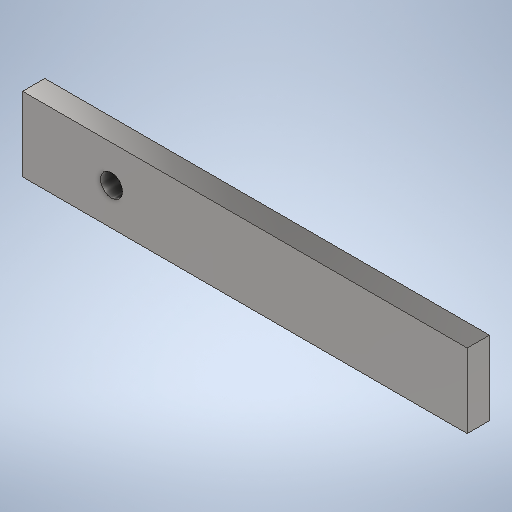
# Autodesk Inventor part: Деталь3
Saved by Autodesk Inventor 2025.1 (Build 291241000, 241)
## iProperties
Created: 2025-04-12
Part Number: Деталь3
Material: Сталь, литейная
Document SubType Name: Modeling
Designer: tishk
Density: 7.85 g/cm^3
Appearance: С умеренной полировкой
Author: tishk
Autodesk Inventor part; units mm, degrees
ref_plane "YZ Plane" through (0, 0, 0) normal (1, 0, 0) x (0, 1, 0)
ref_plane "XZ Plane" through (0, 0, 0) normal (0, 1, 0) x (-1, 0, 0)
ref_plane "XY Plane" through (0, 0, 0) normal (0, 0, 1) x (1, 0, 0)
sketch "Эскиз1" plane through (0, 0, 0) normal (0, 0, 1) x (1, 0, 0)
  line L0 (300, -50) -> (-300, -50)
  line L1 (-300, -50) -> (-300, 50)
  line L2 (-300, 50) -> (300, 50)
  line L3 (300, 50) -> (300, -50)
  line L4 (300, -50) -> (-300, 50) construction
  line L5 (-300, -50) -> (300, 50) construction
  circle A0 centre (-180, 0) radius 15
  point P0 (0, 0)
  dimension "d0" = 100
  dimension "d1" = 600
  dimension "d4" = 30
  dimension "d5" = 120
  constraints: 12 end point, 2 midpoint, 2 parallel, 1 centre point, 1 horizontal, 1 perpendicular
  measures "d0" distance of L2.end L0.start
  measures "d1" distance of L1.end L2.end
  measures "d4" diameter of A0
  measures "d5" distance from line of L1 A0.centre
extrude "Выдавливание1" add sketch "Эскиз1" along normal blind 30
